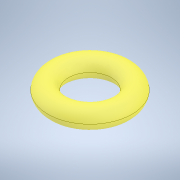
# Autodesk Inventor part: ToeSilikoneRubberStressed
Saved by Autodesk Inventor 2022.2 (Build 262287030, 287C)
## iProperties
Created: 2018-07-16
Part Number: ToeSilikoneRubberStressed
Material: Generic
Document SubType Name: Modeling
Designer: Jochen
Density: 1 g/cm^3
Appearance: Default
Sending System: SolidWorks 2017
Last Author: Felix
Last Saved: 2021-02-23
Author: Jochen
Autodesk Inventor part; units mm, degrees
ref_plane "YZ Plane" through (0, 0, 0) normal (1, 0, 0) x (0, 1, 0)
ref_plane "XZ Plane" through (0, 0, 0) normal (0, 1, 0) x (-1, 0, 0)
ref_plane "XY Plane" through (0, 0, 0) normal (0, 0, 1) x (1, 0, 0)
sketch "Sketch1" plane through (0, 0, 0) normal (1, 0, 0) x (0, 1, 0)
  line L0 (0, -14.7) -> (0, 2.45) construction
  line L1 (-4.5, 0) -> (4.25, 0) construction
  circle A0 centre (0, -9.25) radius 3
  circle A1 centre (0, -9.25) radius 2
  line L2 (2.958, -8.75) -> (-2.958, -8.75) construction
  circle A2 centre (-0.25, -9.25) radius 3
  line L3 (0, -9.25) -> (-0.25, -9.25) construction
  point P0 (0, 0)
  point P1 (0, -6.25)
  point P2 (0, -12.25)
  point P3 (-0.25, -12.25)
  point P4 (2.75, -9.25)
  point P5 (-3, -9.25)
  point P6 (-0.125, -12.2474)
  point P7 (-0.125, -6.2526)
  dimension "d0" = 6
  dimension "d2" = 9.25
  dimension "d19" = 4
  dimension "d22" = 0.5
  dimension "d33" = 0.25
  constraints: 7 point on circle, 4 end point, 3 centre point, 3 point on line, 2 horizontal, 1 coincident, 1 equal radius
  measures "d0" diameter of A0
  measures "d2" distance of point (0, 0) A0.centre
  measures "d19" diameter of A1
  measures "d22" distance from line of A0.centre L2
  measures "d33" distance of A0.centre L3.end
revolve "Revolution1" add sketch "Sketch1" angle 360 about axis through (0, -10, 0) along (0, 1, 0) picked at (-0.3954, -11.8728) contours A2 A0 | A1
sketch "Sketch3" plane through (0, 0, 0) normal (0, 1, 0) x (-1, 0, 0)
  line L0 (16.0374, -3.8798) -> (16.0374, 3.8798)
  circle A0 centre (0, 0) radius 16.5
  line L1 (-23.1, 0) -> (23.1, 0) construction
  line L2 (0, -23.1) -> (0, 23.1) construction
  line L3 (16.0374, 3.8798) -> (-16.5, 0)
  line L4 (16.0374, -3.8798) -> (-16.5, 0)
  line L5 (11.3787, -11.9488) -> (-8.25, 14.2894)
  line L6 (4.6586, -15.8287) -> (-8.25, 14.2894)
  line L7 (-4.6586, -15.8287) -> (8.25, 14.2894)
  line L8 (-11.3787, -11.9488) -> (8.25, 14.2894)
  line L9 (-16.0374, -3.8798) -> (16.5, 0)
  line L10 (-16.0374, 3.8798) -> (16.5, 0)
  line L11 (-11.3787, 11.9488) -> (8.25, -14.2894)
  line L12 (-4.6586, 15.8287) -> (8.25, -14.2894)
  line L13 (4.6586, 15.8287) -> (-8.25, -14.2894)
  line L14 (11.3787, 11.9488) -> (-8.25, -14.2894)
  circle A1 centre (0, 0) radius 9
  line L15 (4.9209, 15.806) -> (-7.9877, -14.3121)
  line L16 (-4.9393, 15.849) -> (7.9693, -14.2691)
  point P0 (0, 4.9593)
  point P1 (-4.2949, 2.4796)
  point P2 (-11.3787, 11.9488)
  point P3 (-4.2949, -2.4796)
  point P4 (-16.0374, -3.8798)
  point P5 (-11.3787, -11.9488)
  point P6 (0, -4.9593)
  point P7 (-4.6586, -15.8287)
  point P8 (4.6586, -15.8287)
  point P9 (4.2949, 2.4796)
  point P10 (4.2949, -2.4796)
  point P11 (11.3787, -11.9488)
  point P12 (-1.2199, -2.113)
  point P13 (-1.2199, 2.113)
  point P14 (-2.4399, 0)
  point P15 (2.4399, 0)
  point P16 (1.2199, -2.113)
  point P17 (1.2199, 2.113)
  point P18 (4.2949, 2.4796)
  point P19 (0, 4.9593)
  point P20 (1.2199, 2.113)
  point P21 (-4.2949, -2.4796)
  point P22 (0, -4.9593)
  point P23 (-1.2199, -2.113)
  point P24 (-4.2949, 2.4796)
  point P25 (-1.2199, 2.113)
  point P26 (-2.4399, 0)
  point P27 (2.4399, 0)
  point P28 (4.2949, -2.4796)
  point P29 (1.2199, -2.113)
  point P30 (-6.827, -5.8645)
  point P31 (-8.4923, -2.9801)
  point P32 (1.6653, -8.8446)
  point P33 (-1.6653, -8.8446)
  point P34 (-8.4923, 2.9801)
  point P35 (-6.827, 5.8645)
  point P36 (-1.6653, 8.8446)
  point P37 (1.6653, 8.8446)
  point P38 (6.827, 5.8645)
  point P39 (8.4923, 2.9801)
  point P40 (8.4923, -2.9801)
  point P41 (6.827, -5.8645)
  point P42 (-4.8994, 15.7558)
  point P43 (-1.9155, 8.7938)
  point P44 (1.9155, 8.7938)
  point P45 (4.8994, 15.7558)
  dimension "d14" = 33
  dimension "d15" = 360
  dimension "d16" = 13.6
  dimension "d20" = 18
  dimension "d31" = 0.25
  dimension "d32" = 0.25
  constraints: 34 end point, 5 coincident, 4 point on circle, 2 centre point, 2 parallel, 1 perpendicular, 1 point on line, 41 other
  measures "d14" diameter of A0
  measures "d16" angle of L4 L3
  measures "d20" diameter of A1
  measures "d31" distance between parallel lines of L15 L13
  measures "d32" distance between parallel lines of L16 L12
extrude "Extrusion2" [suppressed]
fillet "Fillet1" [suppressed]
pattern_circular "Circular Pattern1" [suppressed]
combine "Combine1" [suppressed]
fillet "Fillet2" [suppressed]
equation "\"d32\" = d31"
body "Solid1"
body "Solid7"
body "Solid8"
